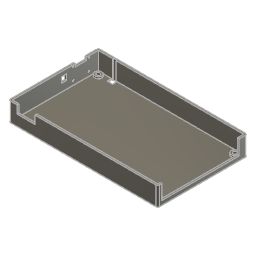
Main Case v15 (Autodesk Fusion 360 design; units mm, degrees)
Autodesk Fusion 360 part; units mm, degrees
note: some values were not read from the file. Set by a fixed rule: which sketch regions a step uses.
sketch "Sketch1" plane through (0, 0, 0) normal (0, 1, 0) x (1, 0, 0)
  line L0 (0, 0) -> (162, 0) construction
  line L1 (162, 0) -> (162, 95) construction
  line L2 (162, 95) -> (0, 95) construction
  line L3 (0, 95) -> (0, 0) construction
  line L4 (4, 91) -> (158, 91) construction
  line L5 (158, 91) -> (158, 4) construction
  line L6 (158, 4) -> (4, 4) construction
  line L7 (4, 4) -> (4, 91) construction
  circle A0 centre (4, 91) radius 2
  circle A1 centre (4, 4) radius 2
  circle A2 centre (158, 4) radius 2
  circle A3 centre (158, 91) radius 2
  line L8 (-1, 96) -> (163, 96)
  line L9 (163, 96) -> (163, -1)
  line L10 (163, -1) -> (-1, -1)
  line L11 (-1, -1) -> (-1, 96)
  line L12 (4, 91) -> (158, 4) construction
  line L13 (162, 95) -> (0, 0) construction
  dimension "d1" = 162
  dimension "d2" = 95
  dimension "d7" = 4
  dimension "d8" = 1
  dimension "d9" = 1
  dimension "d10" = 1
  dimension "d11" = 1
  dimension "d35" = 87
  dimension "d36" = 154
  constraint horizontal L0
  constraint vertical L1
  constraint horizontal L2
  constraint vertical L3
  constraint coincident L0.start L3.end
  constraint horizontal L4
  constraint vertical L5
  constraint horizontal L6
  constraint vertical L7
  constraint coincident L4.start L7.end
  constraint coincident L6.end L7.start
  constraint coincident L5.end L6.start
  constraint coincident L4.end L5.start
  constraint equal A0 A1
  constraint equal A1 A2
  constraint equal A2 A3
  constraint horizontal L8
  constraint vertical L9
  constraint horizontal L10
  constraint vertical L11
  constraint midpoint L12 L13
  measures "d1" distance of L1.end L2.end
  measures "d2" distance of L0.start L2.end
  measures "d7" diameter of A0
  measures "d8" distance of L2 L8
  measures "d9" distance of L1 L9
  measures "d10" distance of L0 L10
  measures "d11" distance of L3 L11
  measures "d35" distance of L4.start L6.end
  measures "d36" distance of L4.start L4.end
extrude "Extrude1" add sketch "Sketch1" along normal blind 1.2
sketch "Sketch2" plane through (0, 1.2, 0) normal (0, 1, 0) x (-1, 0, 0)
  circle A0 centre (-4, -91) radius 2
  circle A1 centre (-158, -4) radius 2
  circle A2 centre (-4, -4) radius 2
  circle A3 centre (-158, -91) radius 2
  line L0 (1, 1) -> (-163, 1)
  line L1 (-163, 1) -> (-163, -96)
  line L2 (-163, -96) -> (1, -96)
  line L3 (1, -96) -> (1, 1)
  circle A4 centre (-4, -91) radius 4
  circle A5 centre (-158, -91) radius 4
  circle A6 centre (-158, -4) radius 4
  circle A7 centre (-4, -4) radius 4
  dimension "d23" = 8
  constraint concentric A0 A4
  constraint concentric A3 A5
  constraint concentric A1 A6
  constraint concentric A2 A7
  constraint equal A4 A7
  constraint equal A4 A5
  constraint equal A5 A6
  measures "d23" diameter of A4
extrude "Extrude2" add sketch "Sketch2" along normal blind 2 contours A4 | A5 | A6 | A7
sketch "Sketch3" plane through (0, 0, 0) normal (0, -1, 0) x (1, 0, 0)
  circle A0 centre (4, -91) radius 2
  circle A1 centre (158, -4) radius 2
  circle A2 centre (4, -4) radius 2
  circle A3 centre (158, -91) radius 2
  line L0 (163, 1) -> (-1, 1)
  line L1 (-1, 1) -> (-1, -96)
  line L2 (-1, -96) -> (163, -96)
  line L3 (163, -96) -> (163, 1)
  line L4 (-1, 1) -> (163, 1)
  line L5 (163, 1) -> (163, -96)
  line L6 (163, -96) -> (-1, -96)
  line L7 (-1, -96) -> (-1, 1)
  line L8 (-3, 3) -> (165, 3)
  line L9 (165, 3) -> (165, -98)
  line L10 (165, -98) -> (-3, -98)
  line L11 (-3, -98) -> (-3, 3)
  dimension "d17" = 2
  dimension "d18" = 2
  dimension "d19" = 2
  dimension "d20" = 2
  constraint horizontal L4
  constraint vertical L5
  constraint horizontal L6
  constraint vertical L7
  constraint coincident L2.end L3.start
  constraint coincident L0.end L1.start
  constraint horizontal L8
  constraint vertical L9
  constraint horizontal L10
  constraint vertical L11
  measures "d17" distance of L4 L8
  measures "d18" distance of L7 L11
  measures "d19" distance of L6 L10
  measures "d20" distance of L5 L9
extrude "Extrude3" add sketch "Sketch3" against normal blind 21.3 contours L8 L9 L10 L11
fillet "Fillet1" radius 2 4 edges at (-3, 10.65, -98) (-3, 10.65, 3) (165, 10.65, 3) (165, 10.65, -98)
sketch "Sketch4" plane through (0, 1.2, 0) normal (0, 1, 0) x (-1, 0, 0)
  circle A0 centre (-4, -4) radius 4
  circle A1 centre (-4, -91) radius 4
  circle A2 centre (-158, -4) radius 4
  circle A3 centre (-158, -91) radius 4
  line L0 (1, 1) -> (-163, 1)
  line L1 (-163, 1) -> (-163, -96)
  line L2 (-163, -96) -> (1, -96)
  line L3 (1, -96) -> (1, 1)
  line L4 (-14, -96) -> (-20, -96)
  line L5 (-20, -96) -> (-20, -91)
  line L6 (-20, -91) -> (-14, -91)
  line L7 (-14, -91) -> (-14, -96)
  dimension "d30" = 6
  dimension "d31" = 5
  dimension "d32" = 15
  constraint horizontal L4
  constraint vertical L5
  constraint horizontal L6
  constraint vertical L7
  constraint coincident L2 L4.end
  measures "d30" distance of L4.start L4.end
  measures "d31" distance of L4.end L5.end
  measures "d32" distance of L2.end L4.start
extrude "Extrude4" cut sketch "Sketch4" against normal up to surface (1.2 mm away) contours L2 L4 L5 L6 L7
sketch "Sketch5" plane through (0, 21.3, 0) normal (0, 1, 0) x (-1, 0, 0)
  arc A0 (-165, -96) -> (-163, -98) centre (-163, -96) ccw
  line L0 (-163, -98) -> (1, -98)
  arc A1 (1, -98) -> (3, -96) centre (1, -96) ccw
  line L1 (3, -96) -> (3, 1)
  arc A2 (3, 1) -> (1, 3) centre (1, 1) ccw
  line L2 (1, 3) -> (-163, 3)
  arc A3 (-163, 3) -> (-165, 1) centre (-163, 1) ccw
  line L3 (-165, 1) -> (-165, -96)
  line L4 (1, -96) -> (-163, -96)
  line L5 (-163, -96) -> (-163, 1)
  line L6 (-163, 1) -> (1, 1)
  line L7 (1, 1) -> (1, -96)
  line L8 (-15, -96) -> (-19, -96)
  line L9 (-19, -96) -> (-19, -96.8)
  line L10 (-19, -96.8) -> (-15, -96.8)
  line L11 (-15, -96.8) -> (-15, -96)
  point P0 (-14, -96)
  dimension "d37" = 4
  dimension "d38" = 1
  dimension "d39" = 0.8
  constraint horizontal L8
  constraint vertical L9
  constraint horizontal L10
  constraint vertical L11
  constraint coincident L4 L8.start
  measures "d37" distance of L9.end L10.end
  measures "d38" distance of L8.start P0
  measures "d39" distance of L8.end L9.end
extrude "Extrude5" cut sketch "Sketch5" against normal up to surface (21.3 mm away) contours L4 L8 L9 L10 L11
sketch "Sketch6" plane through (165, 0, 0) normal (1, 0, 0) x (0, 0, -1)
  line L0 (96, 0) -> (96, 21.3)
  line L1 (96, 21.3) -> (-1, 21.3)
  line L2 (-1, 21.3) -> (-1, 0)
  line L3 (-1, 0) -> (96, 0)
  line L4 (1.7, 21.3) -> (88.7, 21.3)
  line L5 (88.7, 21.3) -> (88.7, 4.8)
  line L6 (88.7, 4.8) -> (1.7, 4.8)
  line L7 (1.7, 4.8) -> (1.7, 21.3)
  dimension "d42" = 2.7
  dimension "d43" = 87
  dimension "d44" = 4.8
  constraint horizontal L4
  constraint vertical L5
  constraint horizontal L6
  constraint vertical L7
  constraint coincident L1 L4.end
  measures "d42" distance of L2 L7
  measures "d43" distance of L4.start L4.end
  measures "d44" distance of L3 L5.end
extrude "Extrude6" cut sketch "Sketch6" against normal up to surface (2 mm away) contours L1 L4 L5 L6 L7
sketch "Sketch7" plane through (-3, 0, 0) normal (-1, 0, 0) x (0, 0, 1)
  line L0 (1, 0) -> (1, 21.3)
  line L1 (1, 21.3) -> (-96, 21.3)
  line L2 (-96, 21.3) -> (-96, 0) construction
  line L3 (-96, 0) -> (1, 0)
  line L4 (-85.5, 20) -> (-67.5, 20) construction
  line L5 (-67.5, 20) -> (-67.5, 6) construction
  line L6 (-67.5, 6) -> (-85.5, 6) construction
  line L7 (-85.5, 6) -> (-85.5, 20) construction
  line L8 (-83, 21.3) -> (-70, 21.3) construction
  line L9 (-70, 21.3) -> (-70, 18.7) construction
  line L10 (-70, 18.7) -> (-83, 18.7) construction
  line L11 (-83, 18.7) -> (-83, 21.3) construction
  line L12 (-83, 21.3) -> (-70, 18.7) construction
  circle A0 centre (-85.5, 20) radius 0.9
  circle A1 centre (-85.5, 6) radius 0.9
  circle A2 centre (-67.5, 6) radius 0.9
  circle A3 centre (-67.5, 20) radius 0.9
  dimension "d47" = 14
  dimension "d48" = 18
  dimension "d51" = 13
  dimension "d52" = 2.6
  dimension "d53" = 26
  dimension "d54" = 1.8
  constraint horizontal L4
  constraint vertical L5
  constraint horizontal L6
  constraint vertical L7
  constraint horizontal L8
  constraint vertical L9
  constraint horizontal L10
  constraint vertical L11
  constraint midpoint L4 L12
  constraint coincident L1 L8.end
  constraint coincident L4.start L7.end
  constraint coincident L6.end L7.start
  constraint coincident L5.end L6.start
  constraint coincident L4.end L5.start
  constraint equal A2 A3
  constraint equal A1 A2
  constraint equal A0 A1
  measures "d47" distance of L4.end L5.end
  measures "d48" distance of L4.start L4.end
  measures "d51" distance of L8.start L8.end
  measures "d52" distance of L8.start L10.end
  measures "d53" distance of L1.end L8.end
  measures "d54" diameter of A0
extrude "Extrude7" cut sketch "Sketch7" against normal up to surface (2 mm away)
sketch "Sketch8" plane through (-3, 0, 0) normal (-1, 0, 0) x (0, 0, 1)
  circle A0 centre (-67.5, 6) radius 0.9
  circle A1 centre (-85.5, 6) radius 0.9
  line L0 (1, 0) -> (1, 21.3)
  line L1 (1, 21.3) -> (-96, 21.3)
  line L2 (-96, 21.3) -> (-96, 0)
  line L3 (-96, 0) -> (1, 0)
  line L4 (-83, 21.3) -> (-70, 21.3)
  line L5 (-70, 21.3) -> (-70, 18.1)
  line L6 (-70, 18.1) -> (-83, 18.1)
  line L7 (-83, 18.1) -> (-83, 21.3)
  point P0 (-83, 21.3)
  point P1 (-70, 21.3)
  dimension "d59" = 3.2
  constraint horizontal L4
  constraint vertical L5
  constraint horizontal L6
  constraint vertical L7
  constraint coincident P0 L4.start
  constraint coincident L5 P1
  measures "d59" distance of P0 L6.end
extrude "Extrude8" cut sketch "Sketch8" against normal up to surface (2 mm away) contours L1 L4 L5 L6 L7
sketch "Sketch9" plane through (-3, 0, 0) normal (-1, 0, 0) x (0, 0, 1)
  line L0 (-83, 18.1) -> (-83, 21.3)
  line L1 (-83, 21.3) -> (-96, 21.3)
  line L2 (-96, 21.3) -> (-96, 0)
  line L3 (-96, 0) -> (1, 0)
  line L4 (1, 0) -> (1, 21.3)
  line L5 (1, 21.3) -> (-70, 21.3)
  line L6 (-70, 21.3) -> (-70, 18.1)
  line L7 (-70, 18.1) -> (-83, 18.1)
  circle A0 centre (-67.5, 20) radius 0.9
  circle A1 centre (-67.5, 6) radius 0.9
  circle A2 centre (-85.5, 20) radius 0.9
  circle A3 centre (-85.5, 6) radius 0.9
  line L8 (-60.2, 16.2) -> (-54.8, 16.2)
  line L9 (-54.8, 16.2) -> (-54.8, 9.8)
  line L10 (-54.8, 9.8) -> (-60.2, 9.8)
  line L11 (-60.2, 9.8) -> (-60.2, 16.2)
  line L12 (-67.5, 20) -> (-67.5, 6) construction
  line L13 (-67.5, 6) -> (-57.5, 13) construction
  line L14 (-57.5, 13) -> (-67.5, 20) construction
  line L15 (-60.2, 16.2) -> (-54.8, 9.8) construction
  dimension "d60" = 6.4
  dimension "d61" = 5.4
  dimension "d62" = 10
  constraint horizontal L8
  constraint vertical L9
  constraint horizontal L10
  constraint vertical L11
  constraint coincident A0.centre L12.start
  constraint coincident A1.centre L12.end
  constraint equal L13 L14
  constraint midpoint L13.end L15
  measures "d60" distance of L8.end L9.end
  measures "d61" distance of L8.start L8.end
  measures "d62" distance of L12 L13.end
extrude "Extrude9" cut sketch "Sketch9" against normal up to surface (2 mm away) contours L8 L9 L10 L11
sketch "Sketch10" plane through (0, 0, 3) normal (0, 0, 1) x (1, 0, 0)
  line L0 (163, 0) -> (163, 21.3)
  line L1 (163, 21.3) -> (-1, 21.3)
  line L2 (-1, 21.3) -> (-1, 0)
  line L3 (-1, 0) -> (163, 0)
  line L4 (6.5, 22.2) -> (26.5, 22.2)
  line L5 (26.5, 22.2) -> (26.5, 12.2)
  line L6 (26.5, 12.2) -> (6.5, 12.2)
  line L7 (6.5, 12.2) -> (6.5, 22.2)
  line L8 (6.5, 22.2) -> (26.5, 12.2) construction
  point P0 (16.5, 17.2)
  dimension "d66" = 20
  dimension "d67" = 10
  dimension "d68" = 17.2
  dimension "d69" = 17.5
  constraint horizontal L4
  constraint vertical L5
  constraint horizontal L6
  constraint vertical L7
  constraint midpoint L8 P0
  measures "d66" distance of L4.start L4.end
  measures "d67" distance of L4.end L5.end
  measures "d68" vertical distance of L2.end P0
  measures "d69" horizontal distance of L1.end P0
extrude "Extrude10" cut sketch "Sketch10" against normal up to surface (2 mm away) contours L1 L5 L6 L7
equation "d21 = -20.00 mm - 1.3 mm"
equation "d42 = 1.7 mm + 1 mm"
equation "d44 = 3.2 mm + 1.6 mm"
equation "d68 = 1.6 mm + 15.6 mm"
